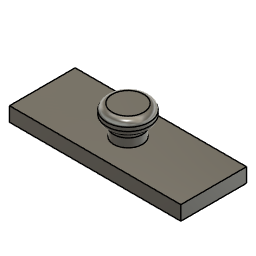
battery cap v1 (Autodesk Fusion 360 design; units mm, degrees)
Autodesk Fusion 360 part; units mm, degrees
sketch "Sketch1" plane through (0, 0, 0) normal (0, 1, 0) x (1, 0, 0)
  line L0 (0, 0) -> (60, 0)
  line L1 (60, 0) -> (60, -23)
  line L2 (60, -23) -> (0, -23)
  line L3 (0, -23) -> (0, 0)
  dimension "d1" = 60
  dimension "d2" = 23
  constraint horizontal L0
  constraint vertical L1
  constraint horizontal L2
  constraint vertical L3
  constraint coincident L0.start L3.end
  measures "d1" distance of L0.start L0.end
  measures "d2" distance of L0.start L2.end
extrude "Extrude1" add sketch "Sketch1" along normal blind 5
sketch "Sketch2" plane through (0, 5, 0) normal (0, 1, 0) x (-1, 0, 0)
  line L0 (0, 23) -> (-60, 23)
  line L1 (-60, 23) -> (-60, 0)
  line L2 (-60, 0) -> (0, 0)
  line L3 (0, 0) -> (0, 23)
  circle A0 centre (-30, 11.5) radius 5
  dimension "d5" = 10
  measures "d5" diameter of A0
extrude "Extrude2" add sketch "Sketch2" along normal blind 5 contours A0
sketch "Sketch3" plane through (0, 10, 0) normal (0, 1, 0) x (-1, 0, 0)
  circle A0 centre (-30, 11.5) radius 5
  circle A1 centre (-30, 11.5) radius 7.5
  dimension "d8" = 15
  constraint concentric A0 A1
  measures "d8" diameter of A1
extrude "Extrude3" add sketch "Sketch3" along normal blind 5 contours A0 | A1
fillet "Fillet1" radius 2 1 edges at (34.6616, 10, 9.6919)
fillet "Fillet2" radius 2 2 edges at (36.9925, 10, 8.7879) (36.9925, 15, 8.7879)
